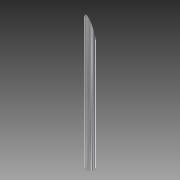
# Autodesk Inventor part: Short_Needle
Saved by Autodesk Inventor 2011 SP2 (Build 150309200, 309)
## iProperties
Created: 2012-02-24
Part Number: Short_Needle
Document SubType Name: Modeling
Designer: sungwook
Density: 1 g/cm^3
Author: sungwook
Autodesk Inventor part; units mm, degrees
ref_plane "YZ Plane" through (0, 0, 0) normal (1, 0, 0) x (0, 1, 0)
ref_plane "XZ Plane" through (0, 0, 0) normal (0, 1, 0) x (-1, 0, 0)
sketch "Sketch1" plane through (0, 0, 0) normal (0, 0, 1) x (1, 0, 0)
  circle A0 centre (0, 0) radius 0.205
  dimension "d0" = 0.41
  constraints: 1 centre point, 1 coincident
  measures "d0" diameter of A0
extrude "Extrusion5" add sketch "Sketch1" along normal blind 7
hole "Hole2" at (0, 0, 0) direction (0, 0, 1) diameter 0.2 end through all
sketch "Sketch10" plane through (0, 0, 0) normal (1, 0, 0) x (0, 1, 0)
  line L0 (0, -1.6) -> (0, 9.6) projected
  line L1 (-0.205, 7) -> (0.205, 7) projected
  line L2 (0.205, 0) -> (0.205, 7) projected
  line L3 (-0.205, 7) -> (0.205, 5.4699)
  line L4 (0.205, 7) -> (-0.205, 7)
  line L5 (0.205, 5.4699) -> (0.205, 7)
  point P0 (0, 0)
  dimension "d52" = 15
  dimension "d53" = 1.5301
  constraints: 6 end point, 2 collinear, 1 point on line
  measures "d52" angle of L5 L3
  measures "d53" distance of L3.end L1.end
extrude "Extrusion6" cut sketch "Sketch10" along normal through all both and the other way through all
ref_plane "Work Plane1" through (0, -0.205, 7) normal (0, 0, -1) x (-1, 0, 0)
body "Solid2"
